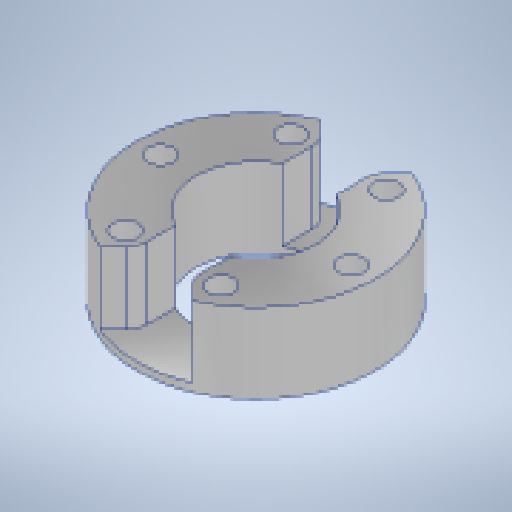
# Autodesk Inventor part: servoplate_forR2_2
Saved by Autodesk Inventor 2024.3 (Build 283343010, 343A)
## iProperties
Created: 2025-05-24
Part Number: servoplate_forR2_2
Material: アルミニウム 6061
Document SubType Name: Modeling
Designer: kshau
Density: 2.7 g/cm^3
Appearance: アルミニウム - フラット
Author: kshau
Autodesk Inventor part; units mm, degrees
ref_plane "YZ Plane" through (0, 0, 0) normal (1, 0, 0) x (0, 1, 0)
ref_plane "XZ Plane" through (0, 0, 0) normal (0, 1, 0) x (-1, 0, 0)
ref_plane "XY Plane" through (0, 0, 0) normal (0, 0, 1) x (1, 0, 0)
sketch "スケッチ1" plane through (0, 0, 0) normal (0, 1, 0) x (-1, 0, 0)
  circle A0 centre (0, 0) radius 15
  dimension "d0" = 30
  constraints: 1 centre point, 1 coincident
  measures "d0" diameter of A0
extrude "押し出し1" add sketch "スケッチ1" along normal blind 10
sketch "スケッチ2" plane through (0, 10, 0) normal (0, 1, 0) x (1, 0, 0)
  circle A0 centre (0, 0) radius 12
  point P0 (-12, 0)
  point P1 (-6, -10.3923)
  point P2 (6, -10.3923)
  point P3 (12, 0)
  point P4 (6, 10.3923)
  point P5 (-6, 10.3923)
  dimension "d3" = 24
  dimension "d6" = 360
  constraints: 1 coincident, 1 horizontal alignment, 9 other
hole "穴1" at (-12, 10, 0) at (-6, 10, 10.3923) at (6, 10, 10.3923) at (12, 10, 0) at (6, 10, -10.3923) at (-6, 10, -10.3923) direction (0, -1, 0) diameter 3.2 end through all
sketch "スケッチ3" plane through (0, 10, 0) normal (0, 1, 0) x (1, 0, 0)
  circle A0 centre (0, 0) radius 7.5
  dimension "d15" = 15
  constraints: 1 centre point, 1 coincident
  measures "d15" diameter of A0
extrude "押し出し2" cut sketch "スケッチ3" against normal blind 10
sketch "スケッチ4" plane through (0, 10, 0) normal (0, 1, 0) x (1, 0, 0)
  circle A0 centre (-6, -10.3923) radius 1.6 projected
  circle A1 centre (6, -10.3923) radius 1.6 projected
  line L0 (-6, -10.3923) -> (6, -10.3923)
  circle A2 centre (-6, -10.3923) radius 2.6
  circle A3 centre (6, -10.3923) radius 2.6
  line L1 (-3.4, -10.3923) -> (-3.4, -6.6851)
  circle A4 centre (0, 0) radius 7.5 projected
  line L2 (3.4, -10.3923) -> (3.4, -6.6851)
  line L3 (-4.1615, -12.2308) -> (-5.7746, -13.8439)
  circle A5 centre (0, 0) radius 15 projected
  line L4 (4.1615, -12.2308) -> (5.7746, -13.8439)
  line L5 (-15, 0) -> (0, 0)
  circle A6 centre (-6, 10.3923) radius 2.6
  circle A7 centre (6, 10.3923) radius 2.6
  line L6 (-3.4, 10.3923) -> (-3.4, 6.6851)
  line L7 (3.4, 10.3923) -> (3.4, 6.6851)
  line L8 (-4.1615, 12.2308) -> (-5.7746, 13.8439)
  line L9 (4.1615, 12.2308) -> (5.7746, 13.8439)
  circle A8 centre (0, 0) radius 7.5
  circle A9 centre (0, 0) radius 15
  dimension "d18" = 1
  dimension "d19" = 1
  dimension "d20" = 135
  constraints: 20 end point, 13 point on circle, 10 symmetric about line, 4 centre point, 4 coincident, 3 tangent, 2 horizontal, 2 point on line, 1 parallel, 1 perpendicular, 1 vertical, 8 other
  measures "d18" radial gap between concentric circles of A0 A2
  measures "d19" radial gap between concentric circles of A1 A3
  measures "d20" angle of L2 L4
extrude "押し出し3" cut sketch "スケッチ4" against normal blind 9 contours L1 A4 L2 L0 | L0 A3 L4 A5 L3 A2 | L6 A6 L8 A5 L9 A7 L7 A4
